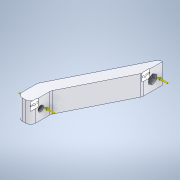
# Autodesk Inventor part: Bottom_Foot_Standoff
Saved by Autodesk Inventor 2021 (Build 250183000, 183)
## iProperties
Created: 2021-10-10
Part Number: Bottom_Foot_Standoff
Material: PET Plastic
Document SubType Name: Modeling
Designer: Jorian Brusind
Density: 1.541 g/cm^3
Appearance: PTFE
Author: Jorian Brusind
Autodesk Inventor part; units mm, degrees
ref_plane "YZ Plane" through (0, 0, 0) normal (1, 0, 0) x (0, 1, 0)
ref_plane "XZ Plane" through (0, 0, 0) normal (0, 1, 0) x (-1, 0, 0)
ref_plane "XY Plane" through (0, 0, 0) normal (0, 0, 1) x (1, 0, 0)
sketch "Sketch1" plane through (0, 0, 0) normal (0, 1, 0) x (-1, 0, 0)
  line L0 (0, 0) -> (-40, 0)
  line L1 (-40, 0) -> (-40, -80)
  line L2 (-40, -80) -> (0, 0)
  line L3 (-41.5, -90) -> (-38.5, -90)
  line L4 (-38.5, -90) -> (-38.5, -70)
  line L5 (-38.5, -70) -> (-41.5, -70)
  line L6 (-41.5, -70) -> (-41.5, -90)
  line L7 (-41.5, -90) -> (-38.5, -70) construction
  line L8 (-38.5, -90) -> (-41.5, -70) construction
  line L9 (1.5, 10) -> (-1.5, 10)
  line L10 (-1.5, 10) -> (-1.5, -10)
  line L11 (-1.5, -10) -> (1.5, -10)
  line L12 (1.5, -10) -> (1.5, 10)
  line L13 (1.5, 10) -> (-1.5, -10) construction
  line L14 (-1.5, 10) -> (1.5, -10) construction
  line L15 (-1.5, 10) -> (-41.5, -70)
  line L16 (1.5, -10) -> (-38.5, -90)
  line L17 (1.5, 10) -> (-11.5, 10)
  line L18 (-11.5, 10) -> (-11.5, -10)
  line L19 (-11.5, -10) -> (1.5, -10)
  line L20 (1.5, -10) -> (1.5, 10)
  dimension "d0" = 40
  dimension "d1" = 80
  dimension "d2" = 3
  dimension "d3" = 20
  dimension "d4" = 3
  dimension "d5" = 20
  dimension "d18" = 20
  constraints: 42 end point, 6 parallel, 4 horizontal, 4 midpoint, 4 perpendicular, 1 point on line
  measures "d0" distance of L0.start L0.end
  measures "d1" distance of L0.end L1.end
  measures "d2" distance of L5.end L4.end
  measures "d3" distance of L4.end L3.end
  measures "d4" distance of L11.end L10.end
  measures "d5" distance of L10.end L9.end
  measures "d18" distance of L18.end L17.end
extrude "Extrusion1" add sketch "Sketch1" along normal blind 20 contours L2 L10 L0 | L0 L10 L9 L12 L11 L2 | L10 L2 L19 L15 L0 | L0 L15 L10 | L10 L19 L2 | L15 L18 L0 | L0 L18 L17 L15 | L19 L11 L16 L4 L2 | L2 L4 L5 L1 L15 L19 | L4 L3 L6 L5 L1 L2 | L2 L1 L5 L4 | L1 L5 L15
sketch "Sketch2" plane through (-1.5, 0, -10) normal (-1, 0, 0) x (0, 0, 1)
  circle A0 centre (10, 10) radius 2.75
  line L0 (0, 0) -> (20, 0) projected
  line L1 (20, 0) -> (20, 20) projected
  point P0 (10, 0)
  dimension "d8" = 5.5
  dimension "d9" = 10
  dimension "d10" = 10
  constraints: 1 centre point
  measures "d8" diameter of A0
  measures "d9" distance from line of L0 A0.centre
  measures "d10" distance from line of L1 A0.centre
sketch "Sketch3" plane through (41.5, 0, -70) normal (1, 0, 0) x (0, 0, -1)
  circle A0 centre (10, 10) radius 2.75
  line L0 (0, 20) -> (20, 20) projected
  line L1 (20, 0) -> (20, 20) projected
  point P0 (-70, 0)
  dimension "d11" = 5.5
  dimension "d12" = 10
  dimension "d13" = 10
  constraints: 1 centre point
  measures "d11" diameter of A0
  measures "d12" distance from line of L0 A0.centre
  measures "d13" distance from line of L1 A0.centre
extrude "Extrusion2" cut sketch "Sketch2" against normal through all
extrude "Extrusion3" cut sketch "Sketch3" against normal through all
sketch "Sketch4" plane through (41.5, 0, -70) normal (1, 0, 0) x (0, 0, -1)
  circle A0 centre (10, 10) radius 2.75 projected
  line L0 (10, 14.6188) -> (14, 12.3094)
  line L1 (14, 12.3094) -> (14, 7.6906)
  line L2 (14, 7.6906) -> (10, 5.3812)
  line L3 (10, 5.3812) -> (6, 7.6906)
  line L4 (6, 7.6906) -> (6, 12.3094)
  line L5 (6, 12.3094) -> (10, 14.6188)
  line L6 (20, 0) -> (20, 20) projected
  point P0 (-70, 0)
  dimension "d19" = 8
  constraints: 12 end point, 1 coincident, 1 parallel, 13 other
  measures "d19" distance between parallel lines of L1 L4
extrude "Extrusion4" cut sketch "Sketch4" against normal blind 4
fillet "Fillet1" radius 5 5 edges at (11.5, 10, -10) (-1.5, 10, -10) (38.5, 10, -90) (11.5, 10, 10) (-1.5, 10, 10)
fillet "Fillet2" radius 5 1 edges at (41.5, 10, -70)
body "Solid1"
